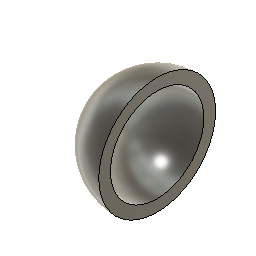
Hip joint Cup (Autodesk Fusion 360 design; units mm, degrees)
Autodesk Fusion 360 part; units mm, degrees
sketch "Sketch1" plane through (0, 0, 0) normal (0, 0, 1) x (1, 0, 0)
sphere "SpherePrimitive1" add diameter 100 placed x (1, 0, 0) y (0, 1, 0) z (0, 0, 1) at (0, 0, 0)
sketch "Sketch2" plane through (0, 0, 0) normal (1, 0, 0) x (0, 1, 0)
  line L0 (75, 50) -> (-75, 50)
  line L1 (-75, 50) -> (-75, -50)
  line L2 (-75, -50) -> (75, -50)
  line L3 (75, -50) -> (75, 50)
  constraint horizontal L0
  constraint vertical L1
  constraint horizontal L2
  constraint vertical L3
extrude "Extrude1" cut sketch "Sketch2" along normal blind 50
shell "Shell1" thickness 10 removed faces 1 at (0, -9.8252, -7.4174)
